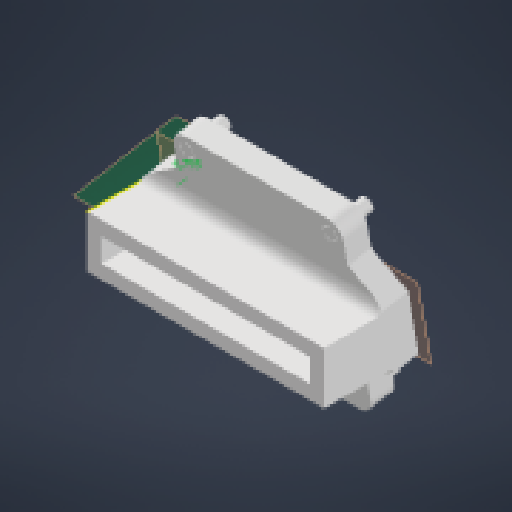
# Autodesk Inventor part: Lock buttom
Saved by Autodesk Inventor 2026.1 (Build 301233020, 233B)
## iProperties
Created: 2025-10-08
Part Number: Lock buttom
Material: Generic
Document SubType Name: Modeling
Designer: Malthe Sennels
Density: 1 g/cm^3
Appearance: Default
Author: Malthe Sennels
Autodesk Inventor part; units mm, degrees
ref_plane "YZ Plane" through (0, 0, 0) normal (1, 0, 0) x (0, 1, 0)
ref_plane "XZ Plane" through (0, 0, 0) normal (0, 1, 0) x (-1, 0, 0)
ref_plane "XY Plane" through (0, 0, 0) normal (0, 0, 1) x (1, 0, 0)
sketch "Sketch1" plane through (0, 0, 0) normal (0, 0, 1) x (1, 0, 0)
  line L0 (0, 0) -> (34, 0)
  line L1 (34, 0) -> (34, 5) construction
  line L2 (0, 5) -> (34, 5)
  line L3 (0, 0) -> (0, 5) construction
  line L4 (39, 0) -> (39, 5)
  line L5 (-5, 0) -> (-5, 5)
  line L6 (0, 5) -> (-5, 5)
  line L7 (39, 5) -> (34, 5)
  line L8 (39, 0) -> (34, 0)
  line L9 (0, 0) -> (-5, 0)
  line L10 (34, 8) -> (0, 8)
  line L11 (0, 8) -> (-8, 8)
  line L12 (-8, 8) -> (-8, -3)
  line L13 (-8, -3) -> (0, -3)
  line L14 (0, -3) -> (34, -3)
  line L15 (34, -3) -> (42, -3)
  line L16 (42, -3) -> (42, 8)
  line L17 (42, 8) -> (34, 8)
extrude "Extrusion1" add sketch "Sketch1" along normal blind 20
ref_plane "Work Plane1" through (-8, -3, 0) normal (0, -0.1736482, 0.9848078) x (1, 0, 0)
sketch "Sketch2" plane through (-8, -3, 0) normal (0, -0.1736482, 0.9848078) x (1, 0, 0)
  line L0 (0, 0) -> (50, 0) projected
  circle A0 centre (40, -10) radius 3
  line L1 (43, -10) -> (43, 0)
  line L2 (37, -10) -> (37, 0)
  circle A1 centre (40, -10) radius 1.5
  line L3 (25, 0) -> (25, -17.6599)
  circle A2 centre (10, -10) radius 3
  line L4 (7, -10) -> (7, 0)
  line L5 (13, -10) -> (13, 0)
  circle A3 centre (10, -10) radius 1.5
  line L6 (37, -5) -> (13, -5)
  line L7 (43, -5) -> (50, 0)
  line L8 (7, -5) -> (0, 0)
  line L9 (47, 2.9544) -> (3, 2.9544) projected
  line L10 (47, 2.9544) -> (50, 2.9544)
  line L11 (50, 2.9544) -> (50, 0)
  line L12 (3, 2.9544) -> (3, 7.8785) projected
  line L13 (3, 2.9544) -> (0, 2.9544)
  line L14 (0, 2.9544) -> (0, 0)
  line L15 (10, -13) -> (40, -13)
  point P0 (8, 2.9544)
  dimension "d4" = 6
  dimension "d5" = 10
  dimension "d6" = 3
  dimension "d7" = 10
  dimension "d8" = 5
  constraints: 26 end point, 6 point on circle, 6 symmetric about line, 5 midpoint, 4 centre point, 4 perpendicular, 3 point on line, 3 tangent, 2 coincident, 1 horizontal, 1 vertical, 2 other
  measures "d4" diameter of A0
  measures "d5" distance from line of L0 A0.centre
  measures "d6" diameter of A1
  measures "d7" horizontal distance of L0.end A0.centre
  measures "d8" distance of L1.end L7.start
extrude "Extrusion2" add sketch "Sketch2" along normal blind 5
sketch "Sketch3" plane through (-8, -3, 0) normal (0, -0.1736482, 0.9848078) x (1, 0, 0)
  line L0 (64.545, 27.5031) -> (-10.6353, 27.5031)
  line L1 (-10.6353, 27.5031) -> (-10.6353, -16.3521)
  line L2 (-10.6353, -16.3521) -> (64.545, -16.3521)
  line L3 (64.545, -16.3521) -> (64.545, 27.5031)
  point P0 (8, 2.9544)
  constraints: 8 end point, 2 parallel, 1 horizontal, 1 perpendicular
extrude "Extrusion3" cut sketch "Sketch3" against normal blind 10
sketch "Sketch4" plane through (-8, -3, 20) normal (-1, 0, 0) x (0, 0, 1)
  line L0 (-18.0604, 11) -> (0, 11) projected
  line L1 (-18.0604, 11) -> (-18.893, 6.2778)
  line L2 (-20.8682, -4.924) -> (-20, 0) projected
  point P0 (-20, 3)
  dimension "d13" = 4.795
  constraints: 2 end point, 1 collinear
  measures "d13" distance of L0.start L1.end
ref_plane "Work Plane4" through (-8, 3.2778, 1.107) normal (0, -0.9848078, -0.1736482) x (1, 0, 0)
sketch "Sketch6" plane through (-8, -3.8682, 4.924) normal (0, -0.1736482, 0.9848078) x (1, 0, 0)
  circle A0 centre (10, -10) radius 1.5 projected
  circle A1 centre (10, -10) radius 1.5
  circle A2 centre (40, -10) radius 1.5 projected
  circle A3 centre (40, -10) radius 1.5
  circle A4 centre (40, -10) radius 1.4
  circle A5 centre (10, -10) radius 1.4
  point P0 (8, 2.9544)
  dimension "d17" = 2.8
  dimension "d18" = 2.8
  constraints: 4 centre point, 4 coincident
  measures "d17" diameter of A4
  measures "d18" diameter of A5
extrude "Extrusion4" add sketch "Sketch6" against normal blind 8 contours A4 | A5
sketch "Sketch8" plane through (-8, -3.8682, 4.924) normal (0, -0.1736482, 0.9848078) x (1, 0, 0)
  circle A0 centre (10, -10) radius 1.5 projected
  circle A1 centre (40, -10) radius 1.5 projected
  circle A2 centre (40, -10) radius 1.5
  circle A3 centre (10, -10) radius 1.5
  point P0 (8, 2.9544)
  constraints: 2 centre point, 2 coincident, 2 concentric
extrude "Extrusion6" add sketch "Sketch8" against normal blind 5
mirror "Mirror3" about plane through (-8, 3.2778, 1.107) normal (0, -0.9848078, -0.1736482) of "Extrusion2", "Extrusion4", "Extrusion6"
fillet "Fillet1" radius 2 2 edges at (17, -3, 5.0771) (17, 8, 7.0167)
body "Solid1"
